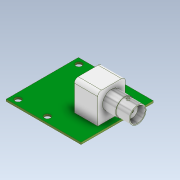
# Autodesk Inventor part: LED8
Saved by Autodesk Inventor 2020 (Build 240168000, 168)
## iProperties
Created: 2020-09-03
Part Number: LED8
Material: Generic
Document SubType Name: Modeling
Designer: Admin
Density: 1 g/cm^3
Appearance: Olive Green
Author: Admin
Autodesk Inventor part; units mm, degrees
ref_plane "YZ Plane" through (0, 0, 0) normal (1, 0, 0) x (0, 1, 0)
ref_plane "XZ Plane" through (0, 0, 0) normal (0, 1, 0) x (-1, 0, 0)
ref_plane "XY Plane" through (0, 0, 0) normal (0, 0, 1) x (1, 0, 0)
sketch "Sketch1" plane through (0, 0, 0) normal (0, 1, 0) x (-1, 0, 0)
  line L0 (0, 0) -> (40, 0)
  line L1 (40, 0) -> (40, -38.6)
  line L2 (40, -38.6) -> (0, -38.6)
  line L3 (0, -38.6) -> (0, 0)
  dimension "d0" = 40
  dimension "d1" = 38.6
  constraints: 8 end point, 2 parallel, 1 horizontal, 1 perpendicular
  measures "d0" distance of L0.start L0.end
  measures "d1" distance of L0.end L1.end
extrude "Extrusion1" add sketch "Sketch1" along normal blind 1
sketch "Sketch6" plane through (0, 1, 0) normal (0, 1, 0) x (1, 0, 0)
  circle A0 centre (-36.676, 3.059) radius 1.6
  circle A1 centre (-21.026, 3.059) radius 1.6
  circle A2 centre (-21.026, 35.541) radius 1.6
  circle A3 centre (-36.676, 35.541) radius 1.6
  line L0 (0, 38.6) -> (-40, 38.6) projected
  line L1 (-40, 38.6) -> (-40, 0) projected
  point P0 (0, 0)
  dimension "d35" = 3.2
  dimension "d36" = 3.2
  dimension "d37" = 3.2
  dimension "d38" = 3.2
  dimension "d39" = 15.65
  dimension "d40" = 15.65
  dimension "d41" = 32.482
  dimension "d42" = 0
  dimension "d43" = 0
  dimension "d44" = 0
  dimension "d45" = 3.059
  dimension "d46" = 3.324
  constraints: 4 centre point
  measures "d35" diameter of A0
  measures "d36" diameter of A1
  measures "d37" diameter of A2
  measures "d38" diameter of A3
  measures "d39" distance of A0.centre A1.centre
  measures "d40" distance of A3.centre A2.centre
  measures "d41" distance of A2.centre A1.centre
  measures "d42" horizontal distance of A2.centre A1.centre
  measures "d43" vertical distance of A1.centre A0.centre
  measures "d44" vertical distance of A2.centre A3.centre
  measures "d45" distance from line of L0 A2.centre
  measures "d46" distance from line of L1 A0.centre
extrude "Extrusion5" cut sketch "Sketch6" against normal blind 5
sketch "Sketch7" plane through (0, 1, 0) normal (0, 1, 0) x (1, 0, 0)
  line L0 (-15.5, 26.65) -> (-3, 26.65)
  line L1 (-3, 26.65) -> (-3, 11.95)
  line L2 (-3, 11.95) -> (-15.5, 11.95)
  line L3 (-15.5, 11.95) -> (-15.5, 26.65)
  line L4 (0, 38.6) -> (-40, 38.6) projected
  line L5 (0, 0) -> (0, 38.6) projected
  dimension "d49" = 12.5
  dimension "d50" = 14.7
  dimension "d51" = 11.95
  dimension "d52" = 3
  constraints: 8 end point, 2 parallel, 1 horizontal, 1 perpendicular
  measures "d49" distance of L0.start L0.end
  measures "d50" distance of L2.end L0.start
  measures "d51" distance between parallel lines of L4 L0
  measures "d52" distance between parallel lines of L5 L1
extrude "Extrusion6" add sketch "Sketch7" along normal blind 15.7
sketch "Sketch9" plane through (-3, 1, -11.95) normal (1, 0, 0) x (0, 0, -1)
  circle A0 centre (7.35, 8.7) radius 4.8
  line L0 (14.7, 0) -> (14.7, 15.7) projected
  line L1 (0, 15.7) -> (14.7, 15.7) projected
  point P0 (-11.95, -1)
  dimension "d55" = 9.6
  dimension "d56" = 7.35
  dimension "d57" = 7
  constraints: 1 centre point
  measures "d55" diameter of A0
  measures "d56" distance from line of L0 A0.centre
  measures "d57" distance from line of L1 A0.centre
extrude "Extrusion7" add sketch "Sketch9" along normal blind 7
fillet "Fillet1" radius 2 2 edges at (-9.25, 16.7, -11.95) (-9.25, 16.7, -26.65)
sketch "Sketch10" plane through (4, 9.7, -19.3) normal (1, 0, 0) x (0, 0, -1)
  circle A0 centre (0, 0) radius 4.5
  line L0 (7.35, -8.7) -> (7.35, 5) projected
  line L1 (-5.35, 7) -> (5.35, 7) projected
  point P0 (-19.3, -9.7)
  dimension "d61" = 9
  dimension "d62" = 7.35
  dimension "d63" = 7
  constraints: 1 centre point
  measures "d61" diameter of A0
  measures "d62" distance from line of L0 A0.centre
  measures "d63" distance from line of L1 A0.centre
extrude "Extrusion8" add sketch "Sketch10" along normal blind 7
sketch "Sketch11" plane through (11, 9.7, -19.3) normal (1, 0, 0) x (0, 0, -1)
  circle A0 centre (0, 0) radius 4
  point P0 (-19.3, -9.7)
  dimension "d66" = 8
  constraints: 1 centre point
  measures "d66" diameter of A0
extrude "Extrusion9" cut sketch "Sketch11" against normal blind 10
sketch "Sketch12" plane through (1, 9.7, -19.3) normal (1, 0, 0) x (0, 0, -1)
  circle A0 centre (0, 0) radius 3.1326
  point P0 (-19.3, -9.7)
  constraints: 1 centre point
extrude "Extrusion10" add sketch "Sketch12" along normal blind 7
sketch "Sketch13" plane through (8, 9.7, -19.3) normal (1, 0, 0) x (0, 0, -1)
  circle A0 centre (0, 0) radius 0.75
  point P0 (-19.3, -9.7)
  dimension "d75" = 1.5
  constraints: 1 centre point
  measures "d75" diameter of A0
extrude "Extrusion11" cut sketch "Sketch13" against normal blind 0.1
sketch "Sketch14" plane through (7.9, 9.7, -19.3) normal (1, 0, 0) x (0, 0, -1)
  circle A0 centre (0, 0) radius 0.2778
  point P0 (-19.3, -9.7)
  constraints: 1 centre point
extrude "Extrusion12" cut sketch "Sketch14" against normal blind 10
sketch "Sketch15" plane through (0, 16.7, 0) normal (0, 1, 0) x (1, 0, 0)
  circle A0 centre (6, 19.3) radius 0.75
  line L0 (-3, 26.65) -> (-15.5, 26.65) projected
  line L1 (-3, 13.95) -> (-3, 24.65) projected
  point P0 (0, 0)
  dimension "d76" = 1.5
  dimension "d77" = 7.35
  dimension "d78" = 9
  constraints: 1 centre point
  measures "d76" diameter of A0
  measures "d77" distance from line of L0 A0.centre
  measures "d78" distance from line of L1 A0.centre
extrude "Extrusion13" add sketch "Sketch15" against normal blind 20
sketch "Sketch16" plane through (6, 16.7, -19.3) normal (0, 1, 0) x (1, 0, 0)
  circle A0 centre (0, 0) radius 0.75
  point P0 (-6, -19.3)
  constraints: 1 centre point
extrude "Extrusion14" cut sketch "Sketch16" against normal blind 1.8
sketch "Sketch17" plane through (6, -3.3, -19.3) normal (0, -1, 0) x (1, 0, 0)
  circle A0 centre (0, 0) radius 0.75
  point P0 (-6, 19.3)
  constraints: 1 centre point
extrude "Extrusion15" cut sketch "Sketch17" against normal blind 7.7
fillet "Fillet2" radius 0.1 1 edges at (5.25, 14.9, -19.3)
body "Solid1"
